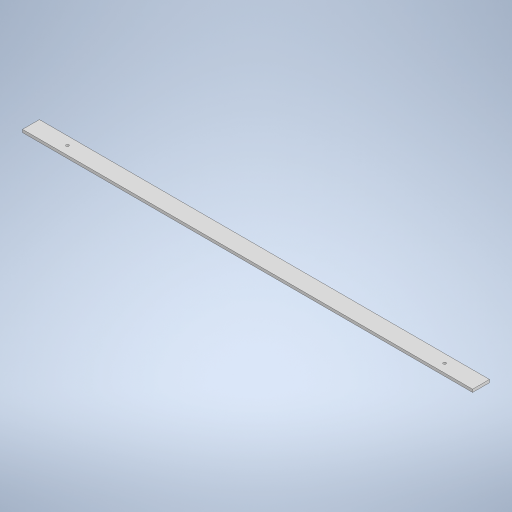
# Autodesk Inventor part: Top Brace
Saved by Autodesk Inventor 2023 (Build 270158000, 158)
## iProperties
Created: 2022-07-27
Part Number: Top Brace
Material: Generic
Document SubType Name: Modeling
Designer: EricPaul
Density: 1 g/cm^3
Appearance: Default
Author: EricPaul
Autodesk Inventor part; units mm, degrees
ref_plane "YZ Plane" through (0, 0, 0) normal (1, 0, 0) x (0, 1, 0)
ref_plane "XZ Plane" through (0, 0, 0) normal (0, 1, 0) x (-1, 0, 0)
ref_plane "XY Plane" through (0, 0, 0) normal (0, 0, 1) x (1, 0, 0)
sketch "Sketch1" plane through (0, 0, 0) normal (0, 1, 0) x (-1, 0, 0)
  line L0 (0, 19.05) -> (1016, 19.05)
  line L1 (1016, 19.05) -> (1016, -19.05)
  line L2 (1016, -19.05) -> (0, -19.05)
  line L3 (0, -19.05) -> (0, 19.05)
  line L4 (0, 19.05) -> (1016, -19.05) construction
  line L5 (1016, 19.05) -> (0, -19.05) construction
  line L6 (1219.2, 0) -> (-203.2, 0) projected
  point P0 (0, 0)
  point P1 (508, 0)
  point P2 (0, 0)
  point P3 (82.296, 0)
  point P4 (933.704, 0)
  dimension "d0" = 1016
  dimension "d1" = 38.1
  dimension "d4" = 82.296
  dimension "d5" = 82.296
  constraints: 12 end point, 3 midpoint, 2 parallel, 2 point on line, 1 coincident, 1 horizontal, 1 perpendicular
  measures "d0" distance of L0.start L0.end
  measures "d1" distance of L0.end L1.end
  measures "d4" distance from line of point (933.704, 0) L1
  measures "d5" distance from line of point (82.296, 0) L3
extrude "Extrusion1" add sketch "Sketch1" along normal blind 6.35
hole "Hole1" at (-933.704, 0, 0) at (-82.296, 0, 0) direction (0, 1, 0) diameter 6.35 end through all
body "Solid1"
